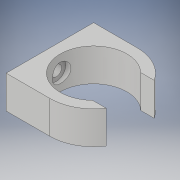
# Autodesk Inventor part: 60mL_falcon_holder
Saved by Autodesk Inventor 2019 (Build 230136000, 136)
## iProperties
Created: 2019-03-07
Part Number: 60mL_falcon_holder
Material: Generic
Document SubType Name: Modeling
Designer: devon
Density: 1 g/cm^3
Appearance: Default
Author: devon
Autodesk Inventor part; units mm, degrees
ref_plane "XZ Plane" through (0, 0, 0) normal (0, 1, 0) x (-1, 0, 0)
ref_plane "XY Plane" through (0, 0, 0) normal (0, 0, 1) x (1, 0, 0)
sketch "Sketch1" plane through (0, 0, 0) normal (0, 1, 0) x (-1, 0, 0)
  circle A0 centre (0, 0) radius 20
  line L0 (0, 20) -> (20, 20)
  line L1 (20, 20) -> (20, -20)
  line L2 (20, -20) -> (0, -20)
  line L3 (0, -20) -> (0, 20)
  dimension "d0" = 40
  constraints: 8 end point, 2 parallel, 1 coincident, 1 horizontal, 1 perpendicular, 1 vertical alignment, 2 other
extrude "Extrusion1" add sketch "Sketch1" along normal blind 15
sketch "Sketch2" plane through (0, 15, 0) normal (0, 1, 0) x (1, 0, 0)
  circle A0 centre (0, 0) radius 15.25
  dimension "d3" = 30.5
  constraints: 1 centre point, 1 coincident
  measures "d3" diameter of A0
extrude "Extrusion2" cut sketch "Sketch2" against normal up to next
sketch "Sketch3" plane through (0, 15, 0) normal (0, 1, 0) x (1, 0, 0)
  line L0 (10, -11) -> (30, -11)
  line L1 (30, -11) -> (30, 11)
  line L2 (30, 11) -> (10, 11)
  line L3 (10, 11) -> (10, -11)
  arc A0 (0, -20) -> (0, 20) centre (0, 0) ccw projected
  line L4 (10, -11) -> (30, 11) construction
  line L5 (30, -11) -> (10, 11) construction
  point P0 (20, 0)
  dimension "d6" = 22
  dimension "d7" = 20
  constraints: 12 end point, 2 midpoint, 2 parallel, 1 horizontal, 1 perpendicular, 1 point on circle
  measures "d6" distance of L2.end L0.start
  measures "d7" distance of L0.start L0.end
extrude "Extrusion3" cut sketch "Sketch3" against normal up to next
ref_plane "Work Plane1" through (-14, 0, 0) normal (1, 0, 0) x (0, 1, 0)
sketch "Sketch7" plane through (-14, 0, 0) normal (1, 0, 0) x (0, 1, 0)
  circle A0 centre (7.5, 0) radius 4.25
  line L0 (0, -15.25) -> (0, 15.25) projected
  point P0 (0, 0)
  point P1 (0, -11)
  point P2 (0, 11)
  dimension "d18" = 8.5
  dimension "d19" = 7.5
  constraints: 1 centre point
  measures "d18" diameter of A0
  measures "d19" distance from line of L0 A0.centre
extrude "Extrusion4" cut sketch "Sketch7" against normal blind 3
sketch "Sketch8" plane through (-17, 7.5, 0) normal (1, 0, 0) x (0, 0, -1)
  circle A0 centre (0, 0) radius 2.375
  point P0 (0, -7.5)
  dimension "d22" = 4.75
  constraints: 1 centre point
  measures "d22" diameter of A0
extrude "Extrusion5" cut sketch "Sketch8" against normal up to next
body "Solid1"
